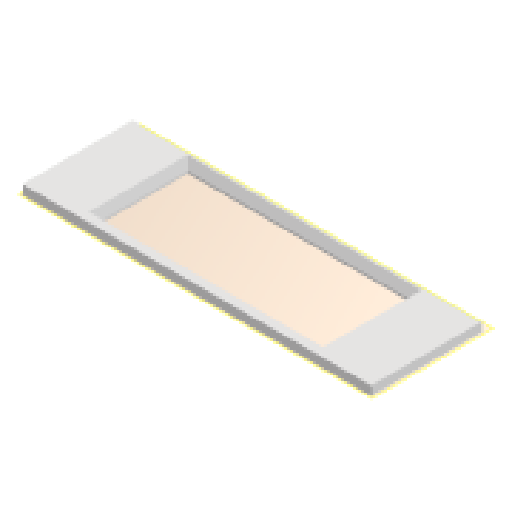
# Autodesk Inventor part: 00_coverglass_frame
Saved by Autodesk Inventor 2024.1 (Build 281209000, 209)
## iProperties
Created: 2024-08-02
Part Number: 00_coverglass_frame
Material: Generisch
Document SubType Name: Modeling
Designer: diederichbenedict
Density: 1 g/cm^3
Appearance: Vorgabe
Author: diederichbenedict
Autodesk Inventor part; units mm, degrees
ref_plane "YZ Plane" through (0, 0, 0) normal (1, 0, 0) x (0, 1, 0)
ref_plane "XZ Plane" through (0, 0, 0) normal (0, 1, 0) x (-1, 0, 0)
ref_plane "XY Plane" through (0, 0, 0) normal (0, 0, 1) x (1, 0, 0)
ref_plane "Arbeitsebene1" through (0, 0, 0) normal (0, 0, 1) x (1, 0, 0)
sketch "Skizze1" plane through (0, 0, 0) normal (0, 0, 1) x (1, 0, 0)
  circle A0 centre (12, 2.9) radius 1.5 projected
  circle A1 centre (-12, 2.9) radius 1.5 projected
  line L0 (38, 12.9) -> (-38, 12.9) projected
  line L1 (38, -12.9) -> (38, 12.9) projected
  line L2 (-38, -12.9) -> (38, -12.9) projected
  line L3 (-38, 12.9) -> (-38, -12.9) projected
  line L4 (-38, -12.9) -> (38, -12.9)
  line L5 (38, -12.9) -> (38, 11.1)
  line L6 (38, 11.1) -> (-38, 11.1)
  line L7 (-38, 11.1) -> (-38, -12.9)
  line L8 (-36, 9.1) -> (36, 9.1)
  line L9 (36, 9.1) -> (36, -10.9)
  line L10 (36, -10.9) -> (-36, -10.9)
  line L11 (-36, -10.9) -> (-36, 9.1)
  line L12 (-36, 9.1) -> (-24, 9.1)
  line L13 (-24, 9.1) -> (-24, -10.9)
  line L14 (-24, -10.9) -> (-36, -10.9)
  line L15 (-36, -10.9) -> (-36, 9.1)
  line L16 (36, 9.1) -> (24, 9.1)
  line L17 (24, 9.1) -> (24, -10.9)
  line L18 (24, -10.9) -> (36, -10.9)
  line L19 (36, -10.9) -> (36, 9.1)
  dimension "d6" = 24
  dimension "d7" = 2
  dimension "d8" = 12
  dimension "d9" = 12
  constraints: 32 end point, 8 parallel, 4 perpendicular, 3 horizontal, 3 point on line, 3 other
  measures "d6" distance of L5.end L4.end
  measures "d7" distance between parallel lines of L6 L8
  measures "d8" distance of L13.end L14.end
  measures "d9" distance of L18.end L17.end
extrude "Extrusion1" add sketch "Skizze1" along normal blind 2 contours L1 L2 L3 L6 | L8 L13 L10 L11 | L8 L9 L10 L17
chamfer "Fasen1" distance 1.5 angle 45 3 edges at (0, 9.1, 2) (24, -0.9, 2) (-24, -0.9, 2)
